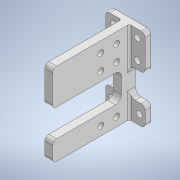
# Autodesk Inventor part: pcb_holder_1
Saved by Autodesk Inventor 2020 (Build 240168000, 168)
## iProperties
Created: 2019-07-22
Part Number: pcb_holder_1
Material: Generic
Document SubType Name: Modeling
Designer: psrob
Density: 1 g/cm^3
Appearance: Default
Author: psrob
Autodesk Inventor part; units mm, degrees
ref_plane "YZ Plane" through (0, 0, 0) normal (1, 0, 0) x (0, 1, 0)
ref_plane "XZ Plane" through (0, 0, 0) normal (0, 1, 0) x (-1, 0, 0)
ref_plane "XY Plane" through (0, 0, 0) normal (0, 0, 1) x (1, 0, 0)
sketch "Sketch1" plane through (0, 0, 0) normal (0, 0, 1) x (1, 0, 0)
  circle A0 centre (6, 16.5583) radius 1.5 projected
  circle A1 centre (7, -6.5583) radius 1.5 projected
  circle A2 centre (7, -26.5583) radius 1.5 projected
  circle A3 centre (15, -36.5583) radius 1.5 projected
  circle A4 centre (15, -16.5583) radius 1.5 projected
  circle A5 centre (14, 16.5583) radius 1.5 projected
  circle A6 centre (6, 26.5583) radius 1.5 projected
  circle A7 centre (14, 36.5583) radius 1.5 projected
  circle A8 centre (15, -6.5583) radius 1.5 projected
  circle A9 centre (15, -26.5583) radius 1.5 projected
  circle A10 centre (7, -36.5583) radius 1.5 projected
  circle A11 centre (7, -16.5583) radius 1.5 projected
  circle A12 centre (14, 26.5583) radius 1.5 projected
  circle A13 centre (6, 36.5583) radius 1.5 projected
  circle A14 centre (-6, 16.5583) radius 1.5 projected
  circle A15 centre (-7, -6.5583) radius 1.5 projected
  circle A16 centre (-7, -26.5583) radius 1.5 projected
  circle A17 centre (-15, -36.5583) radius 1.5 projected
  circle A18 centre (-15, -16.5583) radius 1.5 projected
  circle A19 centre (-14, 16.5583) radius 1.5 projected
  circle A20 centre (-6, 26.5583) radius 1.5 projected
  circle A21 centre (-14, 36.5583) radius 1.5 projected
  circle A22 centre (-15, -6.5583) radius 1.5 projected
  circle A23 centre (-15, -26.5583) radius 1.5 projected
  circle A24 centre (-7, -36.5583) radius 1.5 projected
  circle A25 centre (-7, -16.5583) radius 1.5 projected
  circle A26 centre (-14, 26.5583) radius 1.5 projected
  circle A27 centre (-6, 36.5583) radius 1.5 projected
  circle A28 centre (15.7386, 3.0583) radius 1.5 projected
  circle A29 centre (7.7386, 3.0583) radius 1.5 projected
  circle A30 centre (-15.7386, 3.0583) radius 1.5 projected
  circle A31 centre (-7.7386, 3.0583) radius 1.5 projected
  line L0 (17, 50.5583) -> (20, 47.5583) projected
  line L1 (-17, 50.5583) -> (17, 50.5583) projected
  line L2 (-20, 47.5583) -> (-17, 50.5583) projected
  line L3 (-20, -47.5583) -> (-20, 47.5583) projected
  line L4 (-17, -50.5583) -> (-20, -47.5583) projected
  line L5 (17, -50.5583) -> (-17, -50.5583) projected
  line L6 (20, -47.5583) -> (17, -50.5583) projected
  line L7 (20, 47.5583) -> (20, -47.5583) projected
  circle A32 centre (-7, 46.5583) radius 1.5 projected
  circle A33 centre (-14, 46.5583) radius 1.5 projected
  circle A34 centre (7, 46.5583) radius 1.5 projected
  circle A35 centre (14, 46.5583) radius 1.5 projected
  circle A36 centre (15, -46.5583) radius 1.5 projected
  circle A37 centre (7, -46.5583) radius 1.5 projected
  circle A38 centre (-15, -46.5583) radius 1.5 projected
  circle A39 centre (-7, -46.5583) radius 1.5 projected
  line L8 (6, 16.5583) -> (-6, 16.5583)
  line L9 (-6, 16.5583) -> (-6, 26.5583)
  line L10 (-6, 26.5583) -> (6, 26.5583)
  line L11 (6, 26.5583) -> (6, 16.5583)
  line L12 (6, 16.5583) -> (-6, 26.5583)
  line L13 (-6, 16.5583) -> (6, 26.5583)
  line L14 (10, 12.5583) -> (-10, 12.5583)
  line L15 (-10, 12.5583) -> (-10, 30.5583)
  line L16 (-10, 30.5583) -> (10, 30.5583)
  line L17 (10, 30.5583) -> (10, 12.5583)
  line L18 (10, 12.5583) -> (-10, 30.5583) construction
  line L19 (-10, 12.5583) -> (10, 30.5583) construction
  point P0 (0, 0)
  point P1 (0, 21.5583)
  dimension "d0" = 20
  dimension "d1" = 18
  constraints: 24 end point, 4 midpoint, 4 parallel, 2 horizontal, 2 perpendicular
  measures "d0" distance of L14.start L14.end
  measures "d1" distance of L14.end L15.end
extrude "Extrusion1" add sketch "Sketch1" along normal blind 3 contours A0 L12 L13 A6 L11 | L8 A14 L13 L12 A0 | L13 A14 L9 A20 L12 | L12 A20 L10 A6 L13 | L14 L15 L16 L17
sketch "Sketch2" plane through (0, 0, 3) normal (0, 0, 1) x (1, 0, 0)
  line L0 (10, 12.5583) -> (10, 30.5583) projected
  line L1 (10, 30.5583) -> (-10, 30.5583) projected
  line L2 (-10, 30.5583) -> (-10, 12.5583) projected
  line L3 (-10, 12.5583) -> (10, 12.5583) projected
  circle A0 centre (-6, 16.5583) radius 1.5 projected
  circle A1 centre (6, 16.5583) radius 1.5 projected
  circle A2 centre (-6, 26.5583) radius 1.5 projected
  circle A3 centre (6, 26.5583) radius 1.5 projected
  line L4 (-10, 12.5583) -> (10, 12.5583) projected
  line L5 (0, 12.5583) -> (0, 30.5583)
  line L6 (2, 12.5583) -> (-2, 12.5583)
  line L7 (-2, 12.5583) -> (-2, 30.5583)
  line L8 (-2, 30.5583) -> (2, 30.5583)
  line L9 (2, 30.5583) -> (2, 12.5583)
  line L10 (2, 12.5583) -> (-2, 30.5583) construction
  line L11 (-2, 12.5583) -> (2, 30.5583) construction
  point P0 (0, 0)
  point P1 (0, 21.5583)
  dimension "d4" = 4
  dimension "d5" = 18
  constraints: 14 end point, 5 midpoint, 2 parallel, 1 horizontal, 1 perpendicular
  measures "d4" distance of L6.start L6.end
  measures "d5" distance of L6.end L7.end
ref_plane "Work Plane1" through (3, -21.4417, 25) normal (0, 0, 1) x (1, 0, 0)
extrude "Extrusion2" add sketch "Sketch2" along normal up to surface (22 mm away) contours L3 L5 L1 L9 | L3 L7 L1 L5
sketch "Sketch3" plane through (-2, 12.5583, 3) normal (-1, 0, 0) x (0, 0, 1)
  circle A0 centre (14.5, 12.5) radius 1.5 projected
  circle A1 centre (14.5, 4.5) radius 1.5 projected
  line L0 (19, 21) -> (5, 21) projected
  line L1 (5, 12.5) -> (5, 21) projected
  circle A2 centre (6.5, 12.5) radius 1.5 projected
  line L2 (5, 4.5) -> (5, 12.5) projected
  circle A3 centre (6.5, 4.5) radius 1.5 projected
  line L3 (5, -3.5) -> (5, 4.5) projected
  circle A4 centre (6.5, -3.5) radius 1.5 projected
  line L4 (5, -11.5) -> (5, -3.5) projected
  circle A5 centre (6.5, -11.5) radius 1.5 projected
  line L5 (5, -19.5) -> (5, -11.5) projected
  circle A6 centre (6.5, -19.5) radius 1.5 projected
  line L6 (5, -28) -> (5, -19.5) projected
  line L7 (5, -28) -> (19, -28) projected
  line L8 (19, 21) -> (19, -28) projected
  circle A7 centre (14.5, -19.5) radius 1.5 projected
  circle A8 centre (14.5, -3.5) radius 1.5 projected
  circle A9 centre (14.5, 12.5) radius 1.5 projected
  circle A10 centre (14.5, 4.5) radius 1.5 projected
  circle A11 centre (14.5, -11.5) radius 1.5 projected
  point P0 (-3, -12.5583)
  constraints: 5 horizontal alignment
extrude "Extrusion3" cut sketch "Sketch3" against normal blind 5 contours A0 | A1 | A2 | A3
thicken "Thicken1" operation add thickness 2 both sides no extend neighbours yes toward (0, 0, -1) faces at (-0.6667, 18.5583, 25)
sketch "Sketch4" plane through (0, 0, 3) normal (0, 0, 1) x (1, 0, 0)
  line L0 (-2, 30.5583) -> (2, 30.5583) projected
  line L1 (-2, 12.5583) -> (-2, 30.5583) projected
  line L2 (2, 12.5583) -> (-2, 12.5583) projected
  line L3 (2, 30.5583) -> (2, 12.5583) projected
  line L4 (2, 12.5583) -> (-2, 12.5583)
  line L5 (-2, 12.5583) -> (-2, -1.4417)
  line L6 (-2, -1.4417) -> (2, -1.4417)
  line L7 (2, -1.4417) -> (2, 12.5583)
  line L8 (0, -1.4417) -> (0, -6.4417)
  line L9 (10, -11.4417) -> (10, -1.4417)
  line L10 (10, -1.4417) -> (-10, -1.4417)
  line L11 (-10, -1.4417) -> (-10, -11.4417)
  line L12 (-10, -11.4417) -> (10, -11.4417)
  line L13 (10, -11.4417) -> (-10, -1.4417) construction
  line L14 (10, -1.4417) -> (-10, -11.4417) construction
  circle A0 centre (7, -6.5583) radius 1.5 projected
  line L15 (-6.8625, -18.3992) -> (-6.8625, 36.5158) projected
  circle A1 centre (-7, -6.5583) radius 1.5 projected
  point P0 (0, 0)
  dimension "d12" = 4
  dimension "d13" = 14
  dimension "d14" = 5
  dimension "d15" = 10
  dimension "d16" = 20
  constraints: 22 end point, 5 parallel, 3 midpoint, 2 perpendicular, 1 horizontal, 1 vertical
  measures "d12" distance of L6.end L5.end
  measures "d13" distance of L5.end L4.end
  measures "d14" distance of L8.start L8.end
  measures "d15" distance of L9.start L9.end
  measures "d16" distance of L10.end L9.end
extrude "Extrusion4" add sketch "Sketch4" against normal blind 3 contours L2 L7 L6 L5 | L6 L10 L9 L12 L15 A1 | L15 A1 L12 L11 L10
sketch "Sketch5" plane through (0, 0, 3) normal (0, 0, 1) x (1, 0, 0)
  line L0 (10, -11.4417) -> (10, -1.4417) projected
  line L1 (10, -1.4417) -> (2, -1.4417) projected
  line L2 (2, -1.4417) -> (2, 12.5583) projected
  line L3 (-2, 12.5583) -> (2, 12.5583) projected
  line L4 (-2, 12.5583) -> (-2, -1.4417) projected
  line L5 (-2, -1.4417) -> (-10, -1.4417) projected
  line L6 (-10, -1.4417) -> (-10, -11.4417) projected
  line L7 (-10, -11.4417) -> (10, -11.4417) projected
  circle A0 centre (7, -6.5583) radius 1.5 projected
  circle A1 centre (-7, -6.5583) radius 1.5 projected
  line L8 (-2, -1.4417) -> (-2, 12.5583) projected
  line L9 (-2, -1.4417) -> (2, -1.4417)
  point P0 (0, 0)
  constraints: 2 end point, 1 collinear
extrude "Extrusion5" add sketch "Sketch5" along normal blind 2 contours L9 L4 L3 L2
sketch "Sketch6" plane through (0, 0, 3) normal (0, 0, 1) x (1, 0, 0)
  line L0 (2, -1.4417) -> (-2, -1.4417) projected
  line L1 (-2, -1.4417) -> (-10, -1.4417) projected
  line L2 (-10, -1.4417) -> (-10, -11.4417) projected
  line L3 (-10, -11.4417) -> (10, -11.4417) projected
  line L4 (10, -11.4417) -> (10, -1.4417) projected
  line L5 (10, -1.4417) -> (2, -1.4417) projected
  circle A0 centre (7, -6.5583) radius 1.5 projected
  circle A1 centre (-7, -6.5583) radius 1.5 projected
  line L6 (2, -1.4417) -> (-2, -1.4417)
  line L7 (-2, -1.4417) -> (-2, -11.4417)
  line L8 (-2, -11.4417) -> (2, -11.4417)
  line L9 (2, -11.4417) -> (2, -1.4417)
  point P0 (0, 0)
  constraints: 8 end point, 2 parallel, 1 horizontal, 1 perpendicular, 1 point on line
extrude "Extrusion6" add sketch "Sketch6" along normal up to surface (20 mm away) contours L9 L3 L7 L0
sketch "Sketch7" plane through (-2, 12.5583, 3) normal (-1, 0, 0) x (0, 0, 1)
  circle A0 centre (14.5, -19.5) radius 1.5 projected
  circle A1 centre (6.5, -19.5) radius 1.5 projected
  point P0 (-3, -12.5583)
extrude "Extrusion7" cut sketch "Sketch7" against normal blind 5
fillet "Fillet1" radius 3 6 edges at (-2, -1.4417, 1.5) (-2, 12.5583, 1.5) (2, 12.5583, 1.5) (2, -1.4417, 1.5) (0, 12.5583, 5) (0, -1.4417, 5)
fillet "Fillet2" radius 1 8 edges at (-2, 21.5583, 3) (-2, 11.0583, 3) (-2, -6.4417, 3) (-2, 0.0583, 3) (2, 21.5583, 3) (2, 11.0583, 3) (2, -6.4417, 3) (2, 0.0583, 3)
fillet "Fillet3" radius 2 12 edges at (10, 12.5583, 1.5) (10, -1.4417, 1.5) (10, -11.4417, 1.5) (10, 30.5583, 1.5) (-10, 30.5583, 1.5) (-10, 12.5583, 1.5) (-10, -1.4417, 1.5) (-10, -11.4417, 1.5) (0, -11.4417, 23) (0, -1.4417, 23) (0, 12.5583, 23) (0, 30.5583, 23)
thicken "Thicken2" operation add thickness 2 both sides no extend neighbours yes toward (0, 0, 1) faces at (-0.6667, 6.8916, 5)
thicken "Thicken3" operation add thickness 19 both sides no extend neighbours yes toward (0, 0, 1) faces at (0.6667, 23.8916, 23)
thicken "Thicken4" operation add thickness 19 both sides no extend neighbours yes toward (0, 0, 1) faces at (0.6667, -7.4417, 23)
sketch "Sketch8" plane through (-2, 1.5583, 0) normal (-1, 0, 0) x (0, 0, 1)
  circle A0 centre (36.5, 23.5) radius 1.5 projected
  circle A1 centre (36.5, 15.5) radius 1.5 projected
  circle A2 centre (28.5, 23.5) radius 1.5 projected
  circle A3 centre (28.5, 15.5) radius 1.5 projected
  circle A4 centre (36.5, -8.5) radius 1.5 projected
  circle A5 centre (28.5, -8.5) radius 1.5 projected
  point P0 (0, -1.5583)
extrude "Extrusion8" cut sketch "Sketch8" against normal blind 10
body "Solid1"
